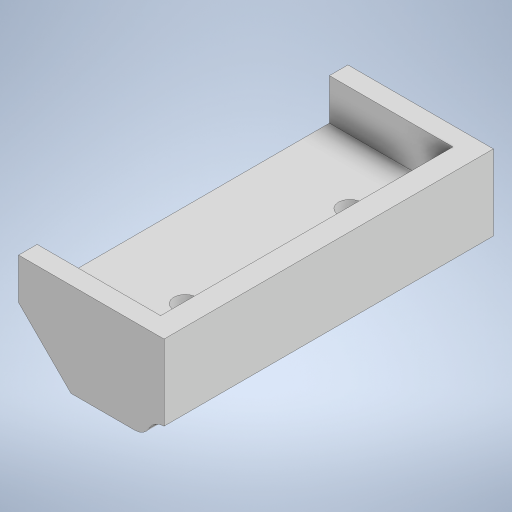
# Autodesk Inventor part: Battery mount bottom
Saved by Autodesk Inventor 2024 (Build 280153000, 153)
## iProperties
Created: 2023-07-25
Part Number: Battery mount bottom
Material: Generic
Document SubType Name: Modeling
Designer: 18179
Density: 1 g/cm^3
Appearance: Default
Author: 18179
Autodesk Inventor part; units mm, degrees
ref_plane "YZ Plane" through (0, 0, 0) normal (1, 0, 0) x (0, 1, 0)
ref_plane "XZ Plane" through (0, 0, 0) normal (0, 1, 0) x (-1, 0, 0)
ref_plane "XY Plane" through (0, 0, 0) normal (0, 0, 1) x (1, 0, 0)
sketch "Sketch1" plane through (0, 0, 0) normal (0, 0, 1) x (1, 0, 0)
  line L0 (0, 0) -> (58.42, 0)
  line L1 (29.21, 0) -> (29.21, -11.176)
  line L2 (0, 0) -> (29.21, 0)
  line L3 (29.21, 0) -> (29.21, -11.176)
  line L4 (29.21, -11.176) -> (0, -11.176)
  line L5 (0, -11.176) -> (0, 0)
  line L6 (0, -11.176) -> (11.176, -11.176)
  line L7 (11.176, -11.176) -> (0, 0)
  line L8 (59.055, 0) -> (29.21, 0)
  line L9 (29.21, 0) -> (29.21, -11.176)
  line L10 (58.42, 0) -> (29.21, 0)
  line L11 (29.21, 0) -> (29.21, -11.176)
  line L12 (29.21, -11.176) -> (50.4337, -11.176)
  line L13 (58.42, -11.176) -> (58.42, -10.16)
  line L14 (58.42, -11.176) -> (90.1357, -11.176)
  line L15 (90.1357, -11.176) -> (90.1357, 0)
  line L16 (90.1357, 0) -> (68.58, 0)
  line L17 (58.42, 0) -> (58.42, -11.176)
  arc A0 (68.58, 0) -> (59.5068, -5.588) centre (68.58, -10.16) ccw
  arc A1 (50.4337, -11.176) -> (59.5068, -5.588) centre (50.4337, -1.016) ccw
  line L18 (58.42, 0) -> (68.58, 0)
  point P0 (58.42, -7.2964)
  dimension "d1" = 11.176
  dimension "d2" = 11.176
  dimension "d3" = 10.16
  dimension "d6" = 68.58
  dimension "d7" = 10.16
  constraints: 38 end point, 6 parallel, 6 point on line, 5 point on circle, 4 tangent, 3 horizontal, 3 perpendicular, 2 centre point, 2 collinear, 1 equal radius, 1 midpoint, 1 vertical
  measures "d1" distance of L1.start L1.end
  measures "d2" distance of L4.end L6.end
  measures "d3" radius of A0
  measures "d6" distance of L0.start L16.end
  measures "d7" radius of A1
extrude "Extrusion1" add sketch "Sketch1" along normal blind 203.2 contours L0 L1 L4 L7 | L0 L17 A1 L12 L1 | L8 L18 A0 A1 L17
sketch "Sketch2" plane through (0, 0, 203.2) normal (0, 0, 1) x (1, 0, 0)
  line L0 (11.176, -11.176) -> (50.4337, -11.176) projected
  line L1 (11.176, -11.176) -> (-21.1529, 21.1529)
  line L2 (0, 0) -> (11.176, -11.176) projected
  line L3 (-21.1529, 21.1529) -> (68.58, 21.1529)
  arc A0 (68.58, 0) -> (59.5068, -5.588) centre (68.58, -10.16) ccw projected
  line L4 (68.58, 21.1529) -> (68.58, 0)
  arc A1 (57.404, 8.0148) -> (49.5263, -0.5588) centre (68.58, -10.16) ccw
  line L5 (57.404, 8.0148) -> (57.404, 9.9769)
  line L6 (5.8283, 9.9769) -> (19.0786, -3.2734)
  line L7 (31.6162, 9.9769) -> (31.6162, 0)
  line L8 (68.58, 0) -> (0, 0) projected
  line L9 (26.0282, 9.9769) -> (26.0282, 0)
  line L10 (37.2042, 9.9769) -> (37.2042, 0)
  point P0 (15.8053, 0)
  point P1 (26.0282, 0)
  point P2 (37.2042, 0)
  point P3 (49.8184, 0)
  dimension "d9" = 45.72
  dimension "d11" = 5.588
  dimension "d12" = 5.588
  constraints: 16 end point, 2 parallel, 2 point on circle, 1 centre point, 1 collinear, 1 horizontal, 1 perpendicular, 1 point on line, 1 vertical, 1 other
  measures "d9" distance of L0.start L1.end
  measures "d11" distance between parallel lines of L7 L9
  measures "d12" distance between parallel lines of L7 L10
extrude "Extrusion2" add sketch "Sketch2" against normal blind 203.2
sketch "Sketch3" plane through (-21.1529, 21.1529, 203.2) normal (0, 1, 0) x (1, 0, 0)
  line L0 (0, 0) -> (0, 203.2) projected
  line L1 (0, 101.6) -> (76.2, 101.6)
  line L2 (76.2, 101.6) -> (76.2, 191.77)
  line L3 (76.2, 191.77) -> (76.2, 11.43)
  line L4 (76.2, 191.77) -> (0, 191.77)
  line L5 (0, 191.77) -> (0, 11.43)
  line L6 (0, 11.43) -> (76.2, 11.43)
  line L7 (76.2, 11.43) -> (76.2, 191.77)
  line L8 (89.7329, 0) -> (0, 0) projected
  line L9 (89.7329, 0) -> (89.7329, 203.2) projected
  line L10 (0, 203.2) -> (89.7329, 203.2) projected
  line L11 (0, 0) -> (0, 203.2) projected
  point P0 (21.1529, 203.2)
  dimension "d15" = 76.2
  dimension "d16" = 90.17
  dimension "d17" = 180.34
  constraints: 14 end point, 2 horizontal, 2 parallel, 2 perpendicular, 2 point on line, 1 midpoint
  measures "d15" distance of L1.start L1.end
  measures "d16" distance of L1.end L2.end
  measures "d17" distance of L2.end L3.end
extrude "Extrusion3" add sketch "Sketch3" along normal blind 25.4 contours L0 L6 L3 L2 L4 L10 L9 L8
sketch "Sketch4" plane through (-21.1529, 21.1529, 11.43) normal (0, 1, 0) x (1, 0, 0)
  line L0 (32.3289, 11.43) -> (71.5866, 11.43) projected
  line L1 (71.5866, 11.43) -> (71.5866, -191.77) projected
  line L2 (32.3289, -191.77) -> (71.5866, -191.77) projected
  line L3 (32.3289, 11.43) -> (32.3289, -191.77) projected
  line L4 (32.3289, -90.17) -> (71.5866, -90.17)
  line L5 (51.9578, -90.17) -> (51.9578, 11.43)
  line L6 (51.9578, -90.17) -> (51.9578, -191.77)
  circle A0 centre (51.9578, -140.97) radius 6.985
  circle A1 centre (51.9578, -39.37) radius 6.985
  point P0 (21.1529, 11.43)
  dimension "d20" = 13.97
  dimension "d21" = 13.97
  constraints: 7 midpoint, 6 end point, 2 centre point
  measures "d20" diameter of A0
  measures "d21" diameter of A1
extrude "Extrusion4" cut sketch "Sketch4" against normal blind 19.05 contours A1 L5 | L5 A1 | A0 L6 | L6 A0
body "Solid1"
